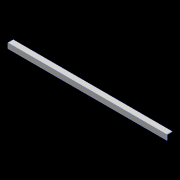
# Autodesk Inventor part: Lbarx2
Saved by Autodesk Inventor 2016 (Build 200138000, 138)
## iProperties
Created: 2019-02-12
Part Number: Lbarx2
Material: Aluminum 6061
Document SubType Name: Modeling
Designer: Calb3e
Density: 2.7 g/cm^3
Appearance: Aluminum - Flat
Author: Calb3e
Autodesk Inventor part; units mm, degrees
ref_plane "YZ Plane" through (0, 0, 0) normal (1, 0, 0) x (0, 1, 0)
ref_plane "XZ Plane" through (0, 0, 0) normal (0, 1, 0) x (-1, 0, 0)
ref_plane "XY Plane" through (0, 0, 0) normal (0, 0, 1) x (1, 0, 0)
sketch "Sketch1" plane through (0, 0, 0) normal (0, 1, 0) x (-1, 0, 0)
  line L0 (0, 0) -> (-600, 0)
  line L1 (-600, 0) -> (-600, -20)
  line L2 (-600, -20) -> (0, -20)
  line L3 (0, -20) -> (0, 0)
  dimension "d0" = 600
  dimension "d1" = 20
  constraints: 8 end point, 2 parallel, 1 horizontal, 1 perpendicular
  measures "d0" distance of L0.start L0.end
  measures "d1" distance of L2.end L0.start
extrude "Extrusion1" add sketch "Sketch1" along normal blind 2
sketch "Sketch2" plane through (0, 2, 0) normal (0, 1, 0) x (1, 0, 0)
  line L0 (0, 0) -> (600, 0)
  line L1 (600, 0) -> (600, 2)
  line L2 (600, 2) -> (0, 2)
  line L3 (0, 2) -> (0, 0)
  dimension "d4" = 600
  dimension "d5" = 2
  constraints: 8 end point, 2 parallel, 1 horizontal, 1 perpendicular
  measures "d4" distance of L2.end L1.end
  measures "d5" distance of L2.end L0.start
extrude "Extrusion2" add sketch "Sketch2" along normal blind 18
body "Solid1"
